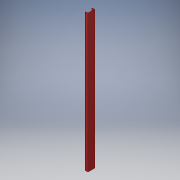
# Autodesk Inventor part: C4 Channel
Saved by Autodesk Inventor 2018.2 (Build 222227000, 227)
## iProperties
Created: 2018-01-22
Part Number: C4 Channel
Material: Steel
Document SubType Name: Modeling
Designer: torba
Density: 7.85 g/cm^3
Appearance: Red
Author: torba
Autodesk Inventor part; units mm, degrees
ref_plane "YZ Plane" through (0, 0, 0) normal (1, 0, 0) x (0, 1, 0)
ref_plane "XZ Plane" through (0, 0, 0) normal (0, 1, 0) x (-1, 0, 0)
ref_plane "XY Plane" through (0, 0, 0) normal (0, 0, 1) x (1, 0, 0)
sketch "Sketch1" plane through (0, 0, 0) normal (0, 1, 0) x (-1, 0, 0)
  line L0 (0, 0) -> (0, -101.6)
  line L1 (0, -101.6) -> (40.2336, -101.6)
  line L2 (40.2336, -101.6) -> (40.2336, 0)
  line L3 (40.2336, 0) -> (0, 0)
  line L4 (0, 0) -> (4.6736, 0)
  line L5 (4.6736, 0) -> (4.6736, -101.6)
  line L6 (4.6736, -101.6) -> (0, -101.6)
  line L7 (0, -101.6) -> (0, 0)
  line L8 (4.6736, 0) -> (40.2336, 0)
  line L9 (40.2336, 0) -> (40.2336, -4.318)
  line L10 (40.2336, -4.318) -> (4.6736, -4.318) construction
  line L11 (4.6736, -4.318) -> (4.6736, 0)
  line L12 (4.6736, -101.6) -> (40.2336, -101.6)
  line L13 (40.2336, -101.6) -> (40.2336, -97.282)
  line L14 (40.2336, -97.282) -> (4.6736, -97.282) construction
  line L15 (4.6736, -97.282) -> (4.6736, -101.6)
  line L16 (4.6736, 0) -> (4.6736, -5.08)
  line L17 (4.6736, -101.6) -> (4.6736, -96.52)
  line L18 (40.2336, -4.318) -> (4.6736, -5.08)
  line L19 (40.2336, -97.282) -> (4.6736, -96.52)
  dimension "d0" = 101.6
  dimension "d1" = 40.2336
  dimension "d2" = 4.6736
  dimension "d3" = 4.318
  dimension "d4" = 4.318
  dimension "d5" = 5.08
  dimension "d6" = 5.08
  constraints: 40 end point, 6 parallel, 6 perpendicular, 5 point on line, 3 horizontal, 1 vertical
  measures "d0" distance of L0.start L0.end
  measures "d1" distance of L0.end L1.end
  measures "d2" distance of L5.end L6.end
  measures "d3" distance of L8.end L9.end
  measures "d4" distance of L13.end L12.end
  measures "d5" distance of L4.end L16.end
  measures "d6" distance of L5.end L17.end
extrude "Extrusion1" add sketch "Sketch1" along normal blind 2057.4 contours L3 L5 L1 L0 | L3 L2 L18 L5 | L5 L19 L2 L1
fillet "Fillet1" radius 3.175 4 edges at (-40.2336, 1028.7, -4.318) (-40.2336, 1028.7, -97.282) (-4.6736, 1028.7, -5.08) (-4.6736, 1028.7, -96.52)
body "Solid1"
